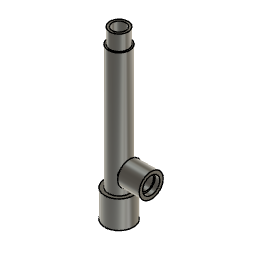
RETHI Vacuum Chamber Material Spring (Autodesk Fusion 360 design; units mm, degrees)
Autodesk Fusion 360 part; units mm, degrees
sketch "Sketch1" plane through (0, 0, 0) normal (0, 0, 1) x (1, 0, 0)
  circle A0 centre (0, 0) radius 4.445
  circle A1 centre (0, 0) radius 6.35
  circle A2 centre (0, 0) radius 2.8575
  dimension "chamberTrack" = 8.89
  dimension "d2" = 12.7
  dimension "chamberDiam" = 5.715
  constraint coincident A0.centre A1.centre
  constraint concentric A0 A2
  measures "chamberTrack" diameter of A0
  measures "d2" diameter of A1
  measures "chamberDiam" diameter of A2
extrude "Extrude1" add sketch "Sketch1" against normal blind 2.54 contours A0
extrude "Extrude2" add sketch "Sketch1" against normal blind 7.62 contours A1
extrude "Extrude3" add sketch "Sketch1" along normal blind 61.9125 contours A0
ref_plane "WorkPlane1" through (4.445, 0, 87.4605) normal (1, 0, 0) x (0, -1, 0)
sketch "Sketch2" plane through (4.445, 0, 87.4605) normal (1, 0, 0) x (0, 1, 0)
  circle A0 centre (0, -76.2) radius 1.905
  circle A1 centre (0, -76.2) radius 3.429
  dimension "d15" = 3.81
  dimension "d95" = 1.524
  measures "d15" diameter of A0
extrude "Extrude4" cut sketch "Sketch2" against normal blind 2.54 contours A0
ref_plane "WorkPlane2" through (0, 0, 56.8325) normal (0, 0, 1) x (1, 0, 0)
sketch "Sketch4" plane through (0, 0, -2.54) normal (0, 0, -1) x (1, 0, 0)
  circle A0 centre (0, 0) radius 2.8575
  circle A1 centre (0, 0) radius 4.445
  circle A2 centre (0, 0) radius 6.35
  circle A3 centre (0, 0) radius 4.445
  constraint coincident A0.centre A1.centre
  constraint concentric A2 A3
extrude "Extrude6" cut sketch "Sketch4" along normal blind 7.62 and the other way blind 2.54 contours A2
sketch "Sketch5" plane through (0, 0, -2.54) normal (0, 0, -1) x (1, 0, 0)
  circle A0 centre (0, 0) radius 2.8575
  circle A1 centre (0, 0) radius 4.445
  circle A2 centre (0, 0) radius 5.95
  circle A3 centre (0, 0) radius 5.4229
  circle A4 centre (0, 0) radius 2.8575
  dimension "bearingInner" = 11.9
  constraint coincident A0.centre A1.centre
  constraint concentric A3 A4
  measures "bearingInner" diameter of A2
extrude "Extrude7" add sketch "Sketch5" against normal blind 6.35 contours A2 | A3
extrude "Extrude8" add 1 faces at (4.8864, 0.4376, -2.54) along direction (0, 0, -1) blind 5.08
sketch "Sketch8" plane through (0, 0, 61.9125) normal (0, 0, 1) x (-1, 0, 0)
  circle A0 centre (0, 0) radius 2.8575
  circle A1 centre (0, 0) radius 4.445
  circle A2 centre (0, 0) radius 3.81
  dimension "d92" = 7.62
  constraint concentric A0 A2
  measures "d92" diameter of A2
extrude "Extrude10" cut sketch "Sketch8" against normal blind 6.35 contours A1
extrude "Extrude11" add sketch "Sketch2" along normal blind 0 and the other way blind 1.5875
sketch "Sketch9" plane through (4.445, 0, 0) normal (1, 0, 0) x (0, 1, 0)
  circle A0 centre (0, 11.2605) radius 1.905
  circle A1 centre (0, 11.2605) radius 5
  circle A2 centre (0, 11.2605) radius 1.905
  arc A3 (0, 14.6895) -> (0, 7.8315) centre (0, 11.2605) ccw
  arc A4 (0, 7.8315) -> (0, 14.6895) centre (0, 11.2605) ccw
  dimension "d100" = 10
  constraint concentric A0 A1
  constraint concentric A1 A2
  measures "d100" diameter of A1
extrude "Extrude12" add sketch "Sketch9" along normal blind 9 contours A1 | A3 A4
sketch "Sketch10" plane through (13.445, 0, 0) normal (1, 0, 0) x (0, 1, 0)
  circle A0 centre (0, 11.2605) radius 1.905
  circle A1 centre (0, 11.2605) radius 5
  circle A2 centre (0, 11.2605) radius 3.585
  circle A3 centre (0, 11.2605) radius 3
  dimension "d103" = 7.17
  dimension "d104" = 6
  constraint concentric A0 A2
  constraint concentric A2 A3
  measures "d103" diameter of A2
  measures "d104" diameter of A3
extrude "Extrude13" cut sketch "Sketch10" against normal blind 2 contours A2
extrude "Extrude14" cut 1 faces at (13.445, 2.6238, 11.1114) along direction (-1, 0, 0) blind 7.62
equation "d2 = chamberTrack + 0.15 in"
equation "chamberDiam = hexDiam + 0.1 in"
equation "hexDiam = 0.125 in"
equation "length = armLength - 1.5 in - 1.5875 mm"
equation "armLength = 4 in"
equation "compressionRoom = 0.3 in"
equation "lipIn = 0.273516 in"
equation "lipOut = 0.305287 in"
